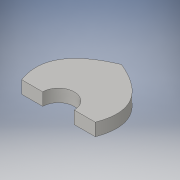
# Autodesk Inventor part: Holder_Side
Saved by Autodesk Inventor 2016 (Build 200138000, 138)
## iProperties
Created: 2018-06-11
Part Number: Holder_Side
Material: Generic
Document SubType Name: Modeling
Designer: Jorian Bruslind
Density: 1 g/cm^3
Appearance: Default
Author: Jorian Bruslind
Autodesk Inventor part; units mm, degrees
ref_plane "YZ Plane" through (0, 0, 0) normal (1, 0, 0) x (0, 1, 0)
ref_plane "XZ Plane" through (0, 0, 0) normal (0, 1, 0) x (-1, 0, 0)
ref_plane "XY Plane" through (0, 0, 0) normal (0, 0, 1) x (1, 0, 0)
sketch "Sketch1" plane through (0, 0, 0) normal (0, 1, 0) x (-1, 0, 0)
  arc A0 (-4.7625, 0) -> (4.7625, 0) centre (0, 0) ccw
  line L0 (4.7625, 0) -> (11.1125, 0)
  line L1 (-4.7625, 0) -> (-11.1125, 0)
  spline S0 degree 2 poles (-11.1125, 0) (-15.8079, -12.4191) (0, -19.05) knots 0 0 0 1 1 1
  spline S1 degree 2 poles (11.1125, 0) (15.8079, -12.4186) (0, -19.05) knots 0 0 0 1 1 1
  point P0 (-4.7625, -10.1621)
  point P1 (4.7625, -10.1621)
  point P2 (-11.1125, -10.1621)
  point P3 (11.1125, -10.1616)
  dimension "d6" = 9.525
  dimension "d7" = 6.35
  dimension "d8" = 6.35
  constraints: 4 end point, 2 horizontal, 2 point on circle, 1 centre point, 6 other
  measures "d6" diameter of A0
  measures "d7" distance of L0.start L0.end
  measures "d8" distance of L1.start L1.end
extrude "Extrusion1" add sketch "Sketch1" along normal blind 3.81
body "Solid1"
